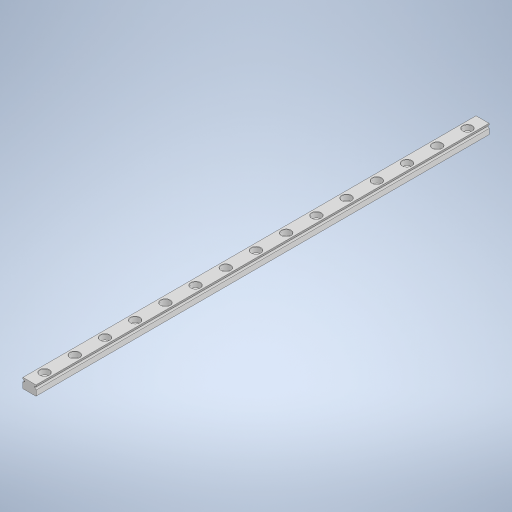
# Autodesk Inventor part: рельса
Saved by Autodesk Inventor 2023.1 (Build 271208000, 208)
## iProperties
Created: 2025-12-22
Part Number: рельса
Material: Типовые
Document SubType Name: Modeling
Designer: DELL
Density: 1 g/cm^3
Appearance: По умолчанию
Author: DELL
Autodesk Inventor part; units mm, degrees
ref_plane "YZ Plane" through (0, 0, 0) normal (1, 0, 0) x (0, 1, 0)
ref_plane "XZ Plane" through (0, 0, 0) normal (0, 1, 0) x (-1, 0, 0)
ref_plane "XY Plane" through (0, 0, 0) normal (0, 0, 1) x (1, 0, 0)
sketch "Эскиз1" plane through (0, 0, 0) normal (0, 0, 1) x (1, 0, 0)
  arc A0 (0.9499, 0.3125) -> (0.1, 0.995) centre (0, 0) ccw projected
  line L0 (0.9499, 0.3125) -> (1.4499, 0.3125) projected
  line L1 (1.4499, 0.3125) -> (1.4499, -0.1875) projected
  line L2 (1.4499, -0.1875) -> (0.9823, -0.1875) projected
  arc A1 (0.1, -0.995) -> (0.9823, -0.1875) centre (0, 0) ccw projected
  line L3 (0.1, -0.995) -> (0.1, -4.5) projected
  line L4 (0.1, -4.5) -> (0.3, -4.7) projected
  line L5 (0.3, -4.7) -> (8.9, -4.7) projected
  line L6 (8.9, -4.7) -> (9.1, -4.5) projected
  line L7 (9.1, -4.5) -> (9.1, -0.995) projected
  arc A2 (8.2177, -0.1875) -> (9.1, -0.995) centre (9.2, 0) ccw projected
  line L8 (8.2177, -0.1875) -> (7.7501, -0.1875) projected
  line L9 (7.7501, -0.1875) -> (7.7501, 0.3125) projected
  line L10 (7.7501, 0.3125) -> (8.2501, 0.3125) projected
  arc A3 (9.1, 0.995) -> (8.2501, 0.3125) centre (9.2, 0) ccw projected
  line L11 (9.1, 0.995) -> (9.1, 1.6) projected
  line L12 (9.1, 1.6) -> (8.9, 1.8) projected
  line L13 (8.9, 1.8) -> (0.3, 1.8) projected
  line L14 (0.3, 1.8) -> (0.1, 1.6) projected
  line L15 (0.1, 1.6) -> (0.1, 0.995) projected
extrude "Выдавливание1" add sketch "Эскиз1" along normal blind 300
sketch "Эскиз2" plane through (0.3, 1.8, 0) normal (0, 1, 0) x (1, 0, 0)
  line L0 (4.3, -2.5) -> (4.3, -42.5) construction
  circle A0 centre (4.3, -10) radius 3
  line L1 (8.6, 0) -> (0, 0) projected
  dimension "d3" = 6
  dimension "d25" = 10
  constraints: 2 end point, 1 centre point, 1 point on line, 1 vertical, 1 other
  measures "d3" diameter of A0
extrude "Выдавливание2" cut sketch "Эскиз2" against normal blind 3.5
sketch "Эскиз3" plane through (0.3, -4.7, 0) normal (0, -1, 0) x (1, 0, 0)
  line L0 (0, 0) -> (8.6, 0) construction
  line L1 (4.3, 0) -> (4.3, 8.2468) construction
  circle A0 centre (4.3, 10) radius 1.75
  point P0 (-0.3, 0)
  dimension "d26" = 3.5
  dimension "d27" = 10
  constraints: 2 end point, 1 centre point, 1 midpoint, 1 point on line, 1 vertical
  measures "d26" diameter of A0
  measures "d27" distance from line of A0.centre L0
extrude "Выдавливание3" cut sketch "Эскиз3" against normal blind 5
chamfer "Фаска1" distance 0.2 angle 45 2 edges at (2.85, -4.7, 10) (1.6, 1.8, 10)
pattern_linear "Прямоуг.массив1" count 15 spacing 20 along (0, 0, 1) of "Выдавливание3", "Выдавливание2", "Фаска1"
